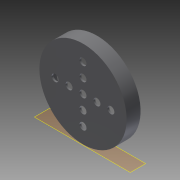
# Autodesk Inventor part: base bund
Saved by Autodesk Inventor 2015 (Build 190159000, 159)
## iProperties
Created: 2017-04-24
Part Number: base bund
Material: ABS Plastic
Document SubType Name: Modeling
Designer: Silas
Density: 1.06 g/cm^3
Appearance: Smooth - White
Author: Silas
Autodesk Inventor part; units mm, degrees
ref_plane "YZ Plane" through (0, 0, 0) normal (1, 0, 0) x (0, 1, 0)
ref_plane "XZ Plane" through (0, 0, 0) normal (0, 1, 0) x (-1, 0, 0)
sketch "Sketch1" plane through (0, 0, 0) normal (0, 1, 0) x (-1, 0, 0)
  circle A0 centre (0, 0) radius 62.5
  dimension "d0" = 125
  constraints: 1 centre point, 1 coincident
  measures "d0" diameter of A0
extrude "Extrusion1" add sketch "Sketch1" along normal blind 20
sketch "Sketch2" plane through (0, 20, 0) normal (0, 1, 0) x (1, 0, 0)
  circle A0 centre (0, 0) radius 60
  dimension "d3" = 120
  constraints: 1 centre point, 1 coincident
  measures "d3" diameter of A0
extrude "Extrusion2" cut sketch "Sketch2" against normal blind 2.5
sketch "Sketch3" plane through (0, 17.5, 0) normal (0, 1, 0) x (1, 0, 0)
  circle A0 centre (0, 0) radius 57.5
  dimension "d6" = 115
  constraints: 1 centre point, 1 coincident
  measures "d6" diameter of A0
extrude "Extrusion3" cut sketch "Sketch3" against normal blind 15
sketch "Sketch4" plane through (0, 2.5, 0) normal (0, 1, 0) x (1, 0, 0)
  circle A0 centre (0, 0) radius 5
  circle A1 centre (0, 20) radius 5
  circle A2 centre (0, 40) radius 5
  circle A3 centre (20, 0) radius 5
  circle A4 centre (40, 0) radius 5
  circle A5 centre (0, -40) radius 5
  circle A6 centre (0, -20) radius 5
  circle A7 centre (-20, 0) radius 5
  circle A8 centre (-40, 0) radius 5
  dimension "d9" = 10
  dimension "d10" = 10
  dimension "d11" = 10
  dimension "d12" = 10
  dimension "d13" = 10
  dimension "d14" = 10
  dimension "d15" = 10
  dimension "d16" = 10
  dimension "d17" = 10
  dimension "d18" = 20
  dimension "d19" = 20
  dimension "d20" = 20
  dimension "d21" = 20
  dimension "d22" = 20
  dimension "d23" = 20
  dimension "d24" = 20
  dimension "d25" = 20
  constraints: 9 centre point, 1 coincident
  measures "d9" diameter of A0
  measures "d10" diameter of A1
  measures "d11" diameter of A2
  measures "d12" diameter of A3
  measures "d13" diameter of A4
  measures "d14" diameter of A5
  measures "d15" diameter of A6
  measures "d16" diameter of A7
  measures "d17" diameter of A8
  measures "d18" distance of A1.centre point (0, 0)
  measures "d19" distance of A2.centre A1.centre
  measures "d20" distance of A3.centre point (0, 0)
  measures "d21" distance of A4.centre A3.centre
  measures "d22" distance of A6.centre point (0, 0)
  measures "d23" distance of A5.centre A6.centre
  measures "d24" distance of point (0, 0) A7.centre
  measures "d25" distance of A8.centre A7.centre
extrude "Extrusion4" cut sketch "Sketch4" against normal up to next
ref_plane "Work Plane1" through (0, 0, -62.5) normal (0, 0, 1) x (1, 0, 0)
sketch "Sketch5" plane through (0, 0, -62.5) normal (0, 0, 1) x (1, 0, 0)
  line L0 (62.5, 20) -> (-62.5, 20) construction
  line L1 (-62.5, 0) -> (62.5, 0) construction
  line L2 (4.25, 10) -> (-4.25, 10)
  line L3 (-4.25, 10) -> (-4.25, 5.5)
  line L4 (-4.25, 5.5) -> (4.25, 5.5)
  line L5 (4.25, 5.5) -> (4.25, 10)
  line L6 (-57.5, 2.5) -> (57.5, 2.5) construction
  line L7 (0, 0) -> (0, 20) construction
  point P0 (0, 5.5)
  dimension "d28" = 8.5
  dimension "d29" = 4.5
  dimension "d61" = 3
  constraints: 10 end point, 2 midpoint, 2 parallel, 1 horizontal, 1 perpendicular, 1 point on line
  measures "d28" distance of L2.start L2.end
  measures "d29" distance of L2.end L3.end
  measures "d61" distance between parallel lines of L6 L4
extrude "Extrusion5" cut sketch "Sketch5" along normal blind 17.5
sketch "Sketch6" plane through (0, 2.5, 0) normal (0, 1, 0) x (1, 0, 0)
  line L0 (0, 0) -> (50, 0) construction
  circle A0 centre (0, 0) radius 5 construction
  line L1 (0, 0) -> (35.3553, -35.3553) construction
  line L2 (0, 0) -> (50, 0) construction
  line L3 (0, 0) -> (0, -50) construction
  line L4 (0, 0) -> (35.3553, 35.3553) construction
  line L5 (0, 0) -> (50, 0) construction
  line L6 (0, 0) -> (0, 50) construction
  line L7 (0, 0) -> (-35.3553, 35.3553) construction
  line L8 (0, 0) -> (50, 0) construction
  line L9 (0, 0) -> (-50, 0) construction
  line L10 (0, 0) -> (50, 0) construction
  line L11 (0, 0) -> (-35.3553, -35.3553) construction
  line L12 (0, 0) -> (50, 0) construction
  circle A1 centre (-35.3553, 35.3553) radius 2
  circle A2 centre (0, 50) radius 2
  circle A3 centre (35.3553, 35.3553) radius 2
  circle A4 centre (50, 0) radius 2
  circle A5 centre (35.3553, -35.3553) radius 2
  circle A6 centre (0, -50) radius 2
  circle A7 centre (-35.3553, -35.3553) radius 2
  circle A8 centre (-50, 0) radius 2
  dimension "d32" = 50
  dimension "d33" = 50
  dimension "d34" = 45
  dimension "d35" = 50
  dimension "d36" = 50
  dimension "d37" = 45
  dimension "d38" = 50
  dimension "d39" = 50
  dimension "d40" = 135
  dimension "d41" = 50
  dimension "d42" = 180
  dimension "d43" = 50
  dimension "d44" = 135
  dimension "d45" = 4
  dimension "d46" = 4
  dimension "d47" = 4
  dimension "d48" = 4
  dimension "d49" = 4
  dimension "d50" = 4
  dimension "d51" = 4
  dimension "d52" = 4
  constraints: 26 end point, 16 coincident, 8 centre point, 7 horizontal, 5 equal length, 1 perpendicular, 1 vertical
  measures "d32" distance of L0.start L0.end
  measures "d33" distance of L1.start L1.end
  measures "d34" angle of L1 L2
  measures "d35" distance of L1.start L3.end
  measures "d36" distance of L1.start L4.end
  measures "d37" angle of L5 L4
  measures "d38" distance of L1.start L6.end
  measures "d39" distance of L1.start L7.end
  measures "d40" angle of L8 L7
  measures "d41" distance of L1.start L9.end
  measures "d42" angle of L9 L10
  measures "d43" distance of L1.start L11.end
  measures "d44" angle of L11 L12
  measures "d45" diameter of A1
  measures "d46" diameter of A2
  measures "d47" diameter of A3
  measures "d48" diameter of A4
  measures "d49" diameter of A5
  measures "d50" diameter of A6
  measures "d51" diameter of A7
  measures "d52" diameter of A8
extrude "Extrusion6" add sketch "Sketch6" along normal blind 17.5 contours A1 | A3 | A4 | A5 | A6 | A7 | A8
sketch "Sketch7" plane through (0, 20, 0) normal (0, 1, 0) x (1, 0, 0)
  circle A0 centre (-35.3553, -35.3553) radius 2 projected
  circle A1 centre (35.3553, -35.3553) radius 2 projected
  circle A2 centre (35.3553, 35.3553) radius 2 projected
  circle A3 centre (-35.3553, 35.3553) radius 2 projected
  circle A4 centre (50, 0) radius 2 projected
  circle A5 centre (0, -50) radius 2 projected
  circle A6 centre (-50, 0) radius 2 projected
  circle A7 centre (0, 0) radius 57.5 projected
  circle A8 centre (0, 40) radius 5 projected
  circle A9 centre (-20, 0) radius 5 projected
  circle A10 centre (0, -40) radius 5 projected
  circle A11 centre (20, 0) radius 5 projected
  circle A12 centre (0, 20) radius 5 projected
  circle A13 centre (0, 0) radius 5 projected
  circle A14 centre (40, 0) radius 5 projected
  circle A15 centre (0, -20) radius 5 projected
  circle A16 centre (-40, 0) radius 5 projected
  circle A17 centre (0, 0) radius 62.5 projected
  line L0 (8.9566, 60) -> (-9.0434, 60)
  line L1 (-9.0434, 60) -> (-9.0434, 17)
  line L2 (-9.0434, 17) -> (8.9566, 17)
  line L3 (8.9566, 17) -> (8.9566, 60)
  line L4 (0, 0) -> (-0.0452, 62.5) construction
  arc A18 (4.25, 62.3553) -> (-4.25, 62.3553) centre (0, 0) ccw construction
  point P0 (-0.0434, 60)
  dimension "d56" = 18
  dimension "d57" = 43
  dimension "d58" = 2.5
  constraints: 10 end point, 2 parallel, 2 point on circle, 1 horizontal, 1 midpoint, 1 perpendicular, 1 point on line
  measures "d56" distance between parallel lines of L1 L3
  measures "d57" distance between parallel lines of L0 L2
  measures "d58" distance from line of L4.end L0
extrude "Extrusion7" cut sketch "Sketch7" against normal up to surface (17.5 mm away) contours L3 L2 A12 L1 A7 | A7 L1 L0 L3 | L2 A12 picked at (-7.6956, 37.9281) picked at (-1.3474, 18.3627)
equation "\"d7\" = d1 - 2 * d4"
equation "\"d10\" = d9"
equation "\"d11\" = d9"
equation "\"d12\" = d9"
equation "\"d13\" = d9"
equation "\"d14\" = d9"
equation "\"d15\" = d9"
equation "\"d16\" = d9"
equation "\"d17\" = d9"
equation "\"d19\" = d18"
equation "\"d20\" = d18"
equation "\"d21\" = d18"
equation "\"d22\" = d18"
equation "\"d23\" = d18"
equation "\"d24\" = d18"
equation "\"d25\" = d18"
equation "\"d33\" = d32"
equation "\"d36\" = d32"
equation "\"d38\" = d32"
equation "\"d39\" = d32"
equation "\"d41\" = d32"
equation "\"d43\" = d32"
equation "\"d46\" = d47"
equation "\"d47\" = d45"
equation "\"d48\" = d45"
equation "\"d49\" = d45"
equation "\"d50\" = d45"
equation "\"d51\" = d45"
equation "\"d52\" = d45"
equation "\"d53\" = d1 - d4"
equation "\"d1\" = 20"
equation "\"d4\" = 2.5"
body "Solid1"
